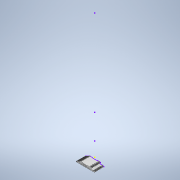
# Autodesk Inventor part: Pieza2
Saved by Autodesk Inventor 2021 (Build 250183000, 183)
## iProperties
Created: 2022-09-12
Part Number: Pieza2
Material: Genérico
Document SubType Name: Chapa
Designer: arthu
Density: 1 g/cm^3
Flat Pattern Width: 60 cm
Flat Pattern Length: 411.221 cm
Flat Pattern Area: 24673.3 cm^2
Sheet Metal Rule: Por defecto
Sheet Metal Width: 600.000 mm
Sheet Metal Length: 4112.213 mm
Sheet Metal Area: 2467327.803 mm^2
Appearance: Valor por defecto
Author: arthu
Autodesk Inventor part; units mm, degrees
(part 1 of 2)
ref_plane "YZ Plane" through (0, 0, 0) normal (1, 0, 0) x (0, 1, 0)
ref_plane "XZ Plane" through (0, 0, 0) normal (0, 1, 0) x (-1, 0, 0)
ref_plane "XY Plane" through (0, 0, 0) normal (0, 0, 1) x (1, 0, 0)
sketch "Boceto1" plane through (0, 0, 0) normal (0, 0, 1) x (1, 0, 0)
  line L0 (593.857, -227.2323) -> (593.8572, -227.2319)
  line L1 (533.5646, -194.9304) -> (533.5644, -194.9308)
  arc A0 (-280.9681, -73.3666) -> (280.9696, -73.3663) centre (0.0001, 907.6925) ccw
  arc A1 (-282.0694, -77.212) -> (282.0709, -77.2117) centre (0.0001, 907.6925) ccw
  line L2 (-378.2765, -109.4682) -> (-318.3462, -77.3608)
  line L3 (-376.3875, -112.9941) -> (-316.4572, -80.8866)
  arc A2 (373.059, -131.7091) -> (376.3889, -112.9936) centre (371.6669, -121.8075) ccw
  arc A3 (373.6159, -135.6702) -> (378.2779, -109.4677) centre (371.6669, -121.8075) ccw
  line L4 (378.2779, -109.4677) -> (318.3477, -77.3604)
  arc A4 (318.3477, -77.3604) -> (280.9696, -73.3663) centre (294.7357, -121.4335) ccw
  arc A5 (316.4587, -80.8863) -> (282.0709, -77.2117) centre (294.7357, -121.4335) ccw
  line L5 (376.3889, -112.9936) -> (316.4587, -80.8863)
  arc A6 (-393.407, -128.772) -> (373.059, -131.7091) centre (-0.011, 2521.9144) ccw
  arc A7 (-393.407, -128.772) -> (-424.3593, -134.1569) centre (-400.7473, -178.2302) ccw
  arc A8 (-393.9943, -132.7287) -> (373.6159, -135.6702) centre (-0.011, 2521.9144) ccw
  arc A9 (-393.9943, -132.7287) -> (-422.4704, -137.6828) centre (-400.7473, -178.2302) ccw
  line L6 (-485.1197, -166.709) -> (-424.3593, -134.1569)
  line L7 (-483.2307, -170.2349) -> (-422.4704, -137.6828)
  arc A10 (-483.2307, -170.2349) -> (-479.0854, -189.0324) centre (-478.5084, -179.0493) ccw
  arc A11 (-485.1197, -166.709) -> (-479.3162, -193.0257) centre (-478.5084, -179.0493) ccw
  arc A12 (-479.3162, -193.0257) -> (508.0847, -191.3269) centre (0.1136, 8102.2313) ccw
  arc A13 (-479.0854, -189.0324) -> (507.8402, -187.3344) centre (0.1136, 8102.2313) ccw
  line L8 (594.8017, -225.469) -> (534.5091, -193.1674)
  line L9 (592.9127, -228.9948) -> (532.6201, -196.6933)
  arc A14 (534.5091, -193.1674) -> (507.8402, -187.3344) centre (510.8969, -237.2409) ccw
  arc A15 (532.6201, -196.6933) -> (508.0847, -191.3269) centre (510.8969, -237.2409) ccw
  line L10 (-588.188, -247.8095) -> (588.1903, -247.8095)
  line L11 (588.1903, -251.8095) -> (400.752, -251.8095)
  arc A16 (588.1903, -247.8095) -> (592.9127, -228.9948) centre (588.1903, -237.8095) ccw
  arc A17 (588.1903, -251.8095) -> (594.8017, -225.469) centre (588.1903, -237.8095) ccw
  line L12 (-588.188, -251.8095) -> (588.1903, -251.8095)
  line L13 (-594.7994, -225.469) -> (-522.4838, -186.7262)
  line L14 (-592.9105, -228.9948) -> (-520.5949, -190.2521)
  arc A18 (-592.9105, -228.9948) -> (-588.188, -247.8095) centre (-588.188, -237.8095) ccw
  arc A19 (-594.7994, -225.469) -> (-588.188, -251.8095) centre (-588.188, -237.8095) ccw
  line L15 (-522.4838, -186.7262) -> (-520.5949, -190.2521)
  line L16 (-378.2765, -109.4682) -> (-376.3875, -112.9941)
  line L17 (0.0011, -247.8095) -> (0.0011, -251.8095)
  line L18 (-483.2307, -170.2349) -> (-485.1197, -166.709)
  line L19 (373.059, -131.7091) -> (373.6159, -135.6702)
  line L20 (268.9094, -80.8863) -> (268.0047, -76.987)
  arc A20 (-282.0694, -77.212) -> (-316.4572, -80.8866) centre (-294.7342, -121.4338) ccw
  arc A21 (-263.5915, -82.3174) -> (-333.7303, -90.1406) centre (-294.7342, -121.4338) ccw
  point P0 (0, 0)
  point P1 (280.9696, -73.3663)
  point P2 (282.0709, -77.2117)
  point P3 (373.059, -131.7091)
  point P4 (-424.3593, -134.1569)
  point P5 (508.0847, -191.3269)
  point P6 (-592.9105, -228.9948)
  point P7 (507.8402, -187.3344)
  point P8 (-422.4704, -137.6828)
  point P9 (378.2779, -109.4677)
  point P10 (-280.9681, -73.3666)
  constraints: 49 point on circle, 42 end point, 22 centre point, 22 tangent, 3 perpendicular, 2 coincident, 2 midpoint, 1 parallel, 1 point on line
extrude "Extrusión1" add sketch "Boceto1" along normal blind 600 contours A0 A4 L4 A3 L19 A2 L5 A5 A1 L20 | A8 A9 L7 L18 L6 A7 A6 L19 | A10 A13 A14 L8 A17 L11 L12 L17 L10 A16 L9 A15 A12 A11 L18 | L12 A19 L13 L15 L14 A18 L10 L17
extrude "Extrusión2" add sketch "Boceto1" along normal blind 600 contours A0 L20 A1 A21 | A21 A1 A20 L3 | A21 L3 L16 L2
sketch "Boceto2" plane through (318.3477, -77.3604, 600) normal (0.4722, 0.8815, 0) x (0.8815, -0.4722, 0)
  line L0 (0, 600) -> (67.989, 600) projected
  line L1 (67.989, 0) -> (81.9881, 0) projected
  line L2 (0, 600) -> (67.989, 600)
  line L3 (67.989, 600) -> (67.989, 0)
  line L4 (67.989, 0) -> (0, 0)
  line L5 (0, 0) -> (0, 600)
  line L6 (0, 600) -> (0, 0) projected
  line L7 (0, 600) -> (0, 300)
  line L8 (0, 300) -> (67.989, 300)
  line L9 (67.989, 600) -> (67.989, 0) projected
  ellipse E0 centre (33.9945, 300) end of major axis (51.9945, 300) minor radius 8
  ellipse E1 centre (33.9945, 332) end of major axis (51.9945, 332) minor radius 8
  ellipse E2 centre (33.9945, 364) end of major axis (51.9945, 364) minor radius 8
  ellipse E3 centre (33.9945, 396) end of major axis (51.9945, 396) minor radius 8
  ellipse E4 centre (33.9945, 428) end of major axis (51.9945, 428) minor radius 8
  ellipse E5 centre (33.9945, 460) end of major axis (51.9945, 460) minor radius 8
  ellipse E6 centre (33.9945, 492) end of major axis (51.9945, 492) minor radius 8
  ellipse E7 centre (33.9945, 524) end of major axis (51.9945, 524) minor radius 8
  ellipse E8 centre (33.9945, 556) end of major axis (51.9945, 556) minor radius 8
  ellipse E9 centre (33.9945, 268) end of major axis (51.9945, 268) minor radius 8
  ellipse E10 centre (33.9945, 300) end of major axis (51.9945, 300) minor radius 8
  ellipse E11 centre (33.9945, 332) end of major axis (51.9945, 332) minor radius 8
  ellipse E12 centre (33.9945, 364) end of major axis (51.9945, 364) minor radius 8
  ellipse E13 centre (33.9945, 396) end of major axis (51.9945, 396) minor radius 8
  ellipse E14 centre (33.9945, 428) end of major axis (51.9945, 428) minor radius 8
  ellipse E15 centre (33.9945, 460) end of major axis (51.9945, 460) minor radius 8
  ellipse E16 centre (33.9945, 492) end of major axis (51.9945, 492) minor radius 8
  ellipse E17 centre (33.9945, 524) end of major axis (51.9945, 524) minor radius 8
  ellipse E18 centre (33.9945, 236) end of major axis (51.9945, 236) minor radius 8
  ellipse E19 centre (33.9945, 268) end of major axis (51.9945, 268) minor radius 8
  ellipse E20 centre (33.9945, 300) end of major axis (51.9945, 300) minor radius 8
  ellipse E21 centre (33.9945, 332) end of major axis (51.9945, 332) minor radius 8
  ellipse E22 centre (33.9945, 364) end of major axis (51.9945, 364) minor radius 8
  ellipse E23 centre (33.9945, 396) end of major axis (51.9945, 396) minor radius 8
  ellipse E24 centre (33.9945, 428) end of major axis (51.9945, 428) minor radius 8
  ellipse E25 centre (33.9945, 460) end of major axis (51.9945, 460) minor radius 8
  ellipse E26 centre (33.9945, 492) end of major axis (51.9945, 492) minor radius 8
  ellipse E27 centre (33.9945, 204) end of major axis (51.9945, 204) minor radius 8
  ellipse E28 centre (33.9945, 236) end of major axis (51.9945, 236) minor radius 8
  ellipse E29 centre (33.9945, 268) end of major axis (51.9945, 268) minor radius 8
  ellipse E30 centre (33.9945, 300) end of major axis (51.9945, 300) minor radius 8
  ellipse E31 centre (33.9945, 332) end of major axis (51.9945, 332) minor radius 8
  ellipse E32 centre (33.9945, 364) end of major axis (51.9945, 364) minor radius 8
  ellipse E33 centre (33.9945, 396) end of major axis (51.9945, 396) minor radius 8
  ellipse E34 centre (33.9945, 428) end of major axis (51.9945, 428) minor radius 8
  ellipse E35 centre (33.9945, 460) end of major axis (51.9945, 460) minor radius 8
  ellipse E36 centre (33.9945, 172) end of major axis (51.9945, 172) minor radius 8
  ellipse E37 centre (33.9945, 204) end of major axis (51.9945, 204) minor radius 8
  ellipse E38 centre (33.9945, 236) end of major axis (51.9945, 236) minor radius 8
  ellipse E39 centre (33.9945, 268) end of major axis (51.9945, 268) minor radius 8
  ellipse E40 centre (33.9945, 300) end of major axis (51.9945, 300) minor radius 8
  ellipse E41 centre (33.9945, 332) end of major axis (51.9945, 332) minor radius 8
  ellipse E42 centre (33.9945, 364) end of major axis (51.9945, 364) minor radius 8
  ellipse E43 centre (33.9945, 396) end of major axis (51.9945, 396) minor radius 8
  ellipse E44 centre (33.9945, 428) end of major axis (51.9945, 428) minor radius 8
  ellipse E45 centre (33.9945, 140) end of major axis (51.9945, 140) minor radius 8
  ellipse E46 centre (33.9945, 172) end of major axis (51.9945, 172) minor radius 8
  ellipse E47 centre (33.9945, 204) end of major axis (51.9945, 204) minor radius 8
  ellipse E48 centre (33.9945, 236) end of major axis (51.9945, 236) minor radius 8
  ellipse E49 centre (33.9945, 268) end of major axis (51.9945, 268) minor radius 8
  ellipse E50 centre (33.9945, 300) end of major axis (51.9945, 300) minor radius 8
  ellipse E51 centre (33.9945, 332) end of major axis (51.9945, 332) minor radius 8
  ellipse E52 centre (33.9945, 364) end of major axis (51.9945, 364) minor radius 8
  ellipse E53 centre (33.9945, 396) end of major axis (51.9945, 396) minor radius 8
  ellipse E54 centre (33.9945, 108) end of major axis (51.9945, 108) minor radius 8
  ellipse E55 centre (33.9945, 140) end of major axis (51.9945, 140) minor radius 8
  ellipse E56 centre (33.9945, 172) end of major axis (51.9945, 172) minor radius 8
  ellipse E57 centre (33.9945, 204) end of major axis (51.9945, 204) minor radius 8
  ellipse E58 centre (33.9945, 236) end of major axis (51.9945, 236) minor radius 8
  ellipse E59 centre (33.9945, 268) end of major axis (51.9945, 268) minor radius 8
  ellipse E60 centre (33.9945, 300) end of major axis (51.9945, 300) minor radius 8
  ellipse E61 centre (33.9945, 332) end of major axis (51.9945, 332) minor radius 8
  ellipse E62 centre (33.9945, 364) end of major axis (51.9945, 364) minor radius 8
  ellipse E63 centre (33.9945, 76) end of major axis (51.9945, 76) minor radius 8
  ellipse E64 centre (33.9945, 108) end of major axis (51.9945, 108) minor radius 8
  ellipse E65 centre (33.9945, 140) end of major axis (51.9945, 140) minor radius 8
  ellipse E66 centre (33.9945, 172) end of major axis (51.9945, 172) minor radius 8
  ellipse E67 centre (33.9945, 204) end of major axis (51.9945, 204) minor radius 8
  ellipse E68 centre (33.9945, 236) end of major axis (51.9945, 236) minor radius 8
  ellipse E69 centre (33.9945, 268) end of major axis (51.9945, 268) minor radius 8
  ellipse E70 centre (33.9945, 300) end of major axis (51.9945, 300) minor radius 8
  ellipse E71 centre (33.9945, 332) end of major axis (51.9945, 332) minor radius 8
  ellipse E72 centre (33.9945, 44) end of major axis (51.9945, 44) minor radius 8
  ellipse E73 centre (33.9945, 76) end of major axis (51.9945, 76) minor radius 8
  ellipse E74 centre (33.9945, 108) end of major axis (51.9945, 108) minor radius 8
  ellipse E75 centre (33.9945, 140) end of major axis (51.9945, 140) minor radius 8
  ellipse E76 centre (33.9945, 172) end of major axis (51.9945, 172) minor radius 8
  ellipse E77 centre (33.9945, 204) end of major axis (51.9945, 204) minor radius 8
  ellipse E78 centre (33.9945, 236) end of major axis (51.9945, 236) minor radius 8
  ellipse E79 centre (33.9945, 268) end of major axis (51.9945, 268) minor radius 8
  ellipse E80 centre (33.9945, 300) end of major axis (51.9945, 300) minor radius 8
  line L10 (245.2285, 600) -> (221.0671, 600) projected
  line L11 (313.6287, 600) -> (313.6287, 0) projected
  line L12 (245.2285, 600) -> (313.6287, 600)
  line L13 (313.6287, 600) -> (313.6287, 0)
  line L14 (313.6287, 0) -> (245.2285, 0)
  line L15 (245.2285, 0) -> (245.2285, 600)
  line L16 (245.2285, 600) -> (245.2285, 0) projected
  line L17 (245.2285, 300) -> (313.6287, 300)
  ellipse E81 centre (279.4286, 300) end of major axis (297.4286, 300) minor radius 8
  ellipse E82 centre (279.4286, 332) end of major axis (297.4286, 332) minor radius 8
  ellipse E83 centre (279.4286, 364) end of major axis (297.4286, 364) minor radius 8
  ellipse E84 centre (279.4286, 396) end of major axis (297.4286, 396) minor radius 8
  ellipse E85 centre (279.4286, 428) end of major axis (297.4286, 428) minor radius 8
  ellipse E86 centre (279.4286, 460) end of major axis (297.4286, 460) minor radius 8
  ellipse E87 centre (279.4286, 492) end of major axis (297.4286, 492) minor radius 8
  ellipse E88 centre (279.4286, 524) end of major axis (297.4286, 524) minor radius 8
  ellipse E89 centre (279.4286, 556) end of major axis (297.4286, 556) minor radius 8
  ellipse E90 centre (279.4286, 268) end of major axis (297.4286, 268) minor radius 8
  ellipse E91 centre (279.4286, 300) end of major axis (297.4286, 300) minor radius 8
  ellipse E92 centre (279.4286, 332) end of major axis (297.4286, 332) minor radius 8
  ellipse E93 centre (279.4286, 364) end of major axis (297.4286, 364) minor radius 8
  ellipse E94 centre (279.4286, 396) end of major axis (297.4286, 396) minor radius 8
  ellipse E95 centre (279.4286, 428) end of major axis (297.4286, 428) minor radius 8
  ellipse E96 centre (279.4286, 460) end of major axis (297.4286, 460) minor radius 8
  ellipse E97 centre (279.4286, 492) end of major axis (297.4286, 492) minor radius 8
  ellipse E98 centre (279.4286, 524) end of major axis (297.4286, 524) minor radius 8
  ellipse E99 centre (279.4286, 236) end of major axis (297.4286, 236) minor radius 8
  ellipse E100 centre (279.4286, 268) end of major axis (297.4286, 268) minor radius 8
  ellipse E101 centre (279.4286, 300) end of major axis (297.4286, 300) minor radius 8
  ellipse E102 centre (279.4286, 332) end of major axis (297.4286, 332) minor radius 8
  ellipse E103 centre (279.4286, 364) end of major axis (297.4286, 364) minor radius 8
  ellipse E104 centre (279.4286, 396) end of major axis (297.4286, 396) minor radius 8
  ellipse E105 centre (279.4286, 428) end of major axis (297.4286, 428) minor radius 8
  ellipse E106 centre (279.4286, 460) end of major axis (297.4286, 460) minor radius 8
  ellipse E107 centre (279.4286, 492) end of major axis (297.4286, 492) minor radius 8
  ellipse E108 centre (279.4286, 204) end of major axis (297.4286, 204) minor radius 8
  ellipse E109 centre (279.4286, 236) end of major axis (297.4286, 236) minor radius 8
  ellipse E110 centre (279.4286, 268) end of major axis (297.4286, 268) minor radius 8
  ellipse E111 centre (279.4286, 300) end of major axis (297.4286, 300) minor radius 8
  ellipse E112 centre (279.4286, 332) end of major axis (297.4286, 332) minor radius 8
  ellipse E113 centre (279.4286, 364) end of major axis (297.4286, 364) minor radius 8
  ellipse E114 centre (279.4286, 396) end of major axis (297.4286, 396) minor radius 8
  ellipse E115 centre (279.4286, 428) end of major axis (297.4286, 428) minor radius 8
  ellipse E116 centre (279.4286, 460) end of major axis (297.4286, 460) minor radius 8
  ellipse E117 centre (279.4286, 172) end of major axis (297.4286, 172) minor radius 8
  ellipse E118 centre (279.4286, 204) end of major axis (297.4286, 204) minor radius 8
  ellipse E119 centre (279.4286, 236) end of major axis (297.4286, 236) minor radius 8
  ellipse E120 centre (279.4286, 268) end of major axis (297.4286, 268) minor radius 8
  ellipse E121 centre (279.4286, 300) end of major axis (297.4286, 300) minor radius 8
  ellipse E122 centre (279.4286, 332) end of major axis (297.4286, 332) minor radius 8
  ellipse E123 centre (279.4286, 364) end of major axis (297.4286, 364) minor radius 8
  ellipse E124 centre (279.4286, 396) end of major axis (297.4286, 396) minor radius 8
  ellipse E125 centre (279.4286, 428) end of major axis (297.4286, 428) minor radius 8
  ellipse E126 centre (279.4286, 140) end of major axis (297.4286, 140) minor radius 8
  ellipse E127 centre (279.4286, 172) end of major axis (297.4286, 172) minor radius 8
  ellipse E128 centre (279.4286, 204) end of major axis (297.4286, 204) minor radius 8
  ellipse E129 centre (279.4286, 236) end of major axis (297.4286, 236) minor radius 8
  ellipse E130 centre (279.4286, 268) end of major axis (297.4286, 268) minor radius 8
  ellipse E131 centre (279.4286, 300) end of major axis (297.4286, 300) minor radius 8
  ellipse E132 centre (279.4286, 332) end of major axis (297.4286, 332) minor radius 8
  ellipse E133 centre (279.4286, 364) end of major axis (297.4286, 364) minor radius 8
  ellipse E134 centre (279.4286, 396) end of major axis (297.4286, 396) minor radius 8
  ellipse E135 centre (279.4286, 108) end of major axis (297.4286, 108) minor radius 8
  ellipse E136 centre (279.4286, 140) end of major axis (297.4286, 140) minor radius 8
  ellipse E137 centre (279.4286, 172) end of major axis (297.4286, 172) minor radius 8
  ellipse E138 centre (279.4286, 204) end of major axis (297.4286, 204) minor radius 8
  ellipse E139 centre (279.4286, 236) end of major axis (297.4286, 236) minor radius 8
  ellipse E140 centre (279.4286, 268) end of major axis (297.4286, 268) minor radius 8
  ellipse E141 centre (279.4286, 300) end of major axis (297.4286, 300) minor radius 8
  ellipse E142 centre (279.4286, 332) end of major axis (297.4286, 332) minor radius 8
  ellipse E143 centre (279.4286, 364) end of major axis (297.4286, 364) minor radius 8
  ellipse E144 centre (279.4286, 76) end of major axis (297.4286, 76) minor radius 8
  ellipse E145 centre (279.4286, 108) end of major axis (297.4286, 108) minor radius 8
  ellipse E146 centre (279.4286, 140) end of major axis (297.4286, 140) minor radius 8
  ellipse E147 centre (279.4286, 172) end of major axis (297.4286, 172) minor radius 8
  ellipse E148 centre (279.4286, 204) end of major axis (297.4286, 204) minor radius 8
  ellipse E149 centre (279.4286, 236) end of major axis (297.4286, 236) minor radius 8
  ellipse E150 centre (279.4286, 268) end of major axis (297.4286, 268) minor radius 8
  ellipse E151 centre (279.4286, 300) end of major axis (297.4286, 300) minor radius 8
  ellipse E152 centre (279.4286, 332) end of major axis (297.4286, 332) minor radius 8
  ellipse E153 centre (279.4286, 44) end of major axis (297.4286, 44) minor radius 8
  ellipse E154 centre (279.4286, 76) end of major axis (297.4286, 76) minor radius 8
  ellipse E155 centre (279.4286, 108) end of major axis (297.4286, 108) minor radius 8
  ellipse E156 centre (279.4286, 140) end of major axis (297.4286, 140) minor radius 8
  ellipse E157 centre (279.4286, 172) end of major axis (297.4286, 172) minor radius 8
  ellipse E158 centre (279.4286, 204) end of major axis (297.4286, 204) minor radius 8
  ellipse E159 centre (279.4286, 236) end of major axis (297.4286, 236) minor radius 8
  ellipse E160 centre (279.4286, 268) end of major axis (297.4286, 268) minor radius 8
  ellipse E161 centre (279.4286, 300) end of major axis (297.4286, 300) minor radius 8
  point P0 (-317.1463, 600)
  point P1 (76.2536, 0)
  point P2 (279.4286, 308)
  point P3 (279.4286, 292)
  point P4 (33.9945, 308)
  point P5 (33.9945, 292)
  point P6 (279.4286, 340)
  point P7 (279.4286, 324)
  point P8 (279.4286, 372)
  point P9 (279.4286, 356)
  point P10 (279.4286, 404)
  point P11 (279.4286, 388)
  point P12 (279.4286, 436)
  point P13 (279.4286, 420)
  point P14 (279.4286, 468)
  point P15 (279.4286, 452)
  point P16 (279.4286, 500)
  point P17 (279.4286, 484)
  point P18 (279.4286, 532)
  point P19 (279.4286, 516)
  point P20 (279.4286, 564)
  point P21 (279.4286, 548)
  point P22 (279.4286, 276)
  point P23 (279.4286, 260)
  point P24 (279.4286, 308)
  point P25 (279.4286, 292)
  point P26 (279.4286, 340)
  point P27 (279.4286, 324)
  point P28 (279.4286, 372)
  point P29 (279.4286, 356)
  point P30 (279.4286, 404)
  point P31 (279.4286, 388)
  point P32 (279.4286, 436)
  point P33 (279.4286, 420)
  point P34 (279.4286, 468)
  point P35 (279.4286, 452)
  point P36 (279.4286, 500)
  point P37 (279.4286, 484)
  point P38 (279.4286, 532)
  point P39 (279.4286, 516)
  point P40 (279.4286, 244)
  point P41 (279.4286, 228)
  point P42 (279.4286, 276)
  point P43 (279.4286, 260)
  point P44 (279.4286, 308)
  point P45 (279.4286, 292)
  point P46 (279.4286, 340)
  point P47 (279.4286, 324)
  point P48 (279.4286, 372)
  point P49 (279.4286, 356)
  point P50 (279.4286, 404)
  point P51 (279.4286, 388)
  point P52 (279.4286, 436)
  point P53 (279.4286, 420)
  point P54 (279.4286, 468)
  point P55 (279.4286, 452)
  point P56 (279.4286, 500)
  point P57 (279.4286, 484)
  point P58 (279.4286, 212)
  point P59 (279.4286, 196)
  point P60 (279.4286, 244)
  point P61 (279.4286, 228)
  point P62 (279.4286, 276)
  point P63 (279.4286, 260)
  point P64 (279.4286, 308)
  point P65 (279.4286, 292)
  point P66 (279.4286, 340)
  point P67 (279.4286, 324)
  point P68 (279.4286, 372)
  point P69 (279.4286, 356)
  point P70 (279.4286, 404)
  point P71 (279.4286, 388)
  point P72 (279.4286, 436)
  point P73 (279.4286, 420)
  point P74 (279.4286, 468)
  point P75 (279.4286, 452)
  point P76 (279.4286, 180)
  point P77 (279.4286, 164)
  point P78 (279.4286, 212)
  point P79 (279.4286, 196)
  point P80 (279.4286, 244)
  point P81 (279.4286, 228)
  point P82 (279.4286, 276)
  point P83 (279.4286, 260)
  point P84 (279.4286, 308)
  point P85 (279.4286, 292)
  point P86 (279.4286, 340)
  point P87 (279.4286, 324)
  point P88 (279.4286, 372)
  point P89 (279.4286, 356)
  point P90 (279.4286, 404)
  point P91 (279.4286, 388)
  point P92 (279.4286, 436)
  point P93 (279.4286, 420)
  point P94 (279.4286, 148)
  point P95 (279.4286, 132)
  point P96 (279.4286, 180)
  point P97 (279.4286, 164)
  point P98 (279.4286, 212)
  point P99 (279.4286, 196)
  point P100 (279.4286, 244)
  point P101 (279.4286, 228)
  point P102 (279.4286, 276)
  point P103 (279.4286, 260)
  point P104 (279.4286, 308)
  point P105 (279.4286, 292)
  point P106 (279.4286, 340)
  point P107 (279.4286, 324)
  point P108 (279.4286, 372)
  point P109 (279.4286, 356)
  point P110 (279.4286, 404)
  point P111 (279.4286, 388)
  point P112 (279.4286, 116)
  point P113 (279.4286, 100)
  point P114 (279.4286, 148)
  point P115 (279.4286, 132)
  point P116 (279.4286, 180)
  point P117 (279.4286, 164)
  point P118 (279.4286, 212)
  point P119 (279.4286, 196)
  point P120 (279.4286, 244)
  point P121 (279.4286, 228)
  point P122 (279.4286, 276)
  point P123 (279.4286, 260)
  point P124 (279.4286, 308)
  point P125 (279.4286, 292)
  point P126 (279.4286, 340)
  point P127 (279.4286, 324)
  point P128 (279.4286, 372)
  point P129 (279.4286, 356)
  point P130 (279.4286, 84)
  point P131 (279.4286, 68)
  point P132 (279.4286, 116)
  point P133 (279.4286, 100)
  point P134 (279.4286, 148)
  point P135 (279.4286, 132)
  point P136 (279.4286, 180)
  point P137 (279.4286, 164)
  point P138 (279.4286, 212)
  point P139 (279.4286, 196)
  point P140 (279.4286, 244)
  point P141 (279.4286, 228)
  point P142 (279.4286, 276)
  point P143 (279.4286, 260)
  point P144 (279.4286, 308)
  point P145 (279.4286, 292)
  point P146 (279.4286, 340)
  point P147 (279.4286, 324)
  point P148 (279.4286, 52)
  point P149 (279.4286, 36)
  point P150 (279.4286, 84)
  point P151 (279.4286, 68)
  point P152 (279.4286, 116)
  point P153 (279.4286, 100)
  point P154 (279.4286, 148)
  point P155 (279.4286, 132)
  point P156 (279.4286, 180)
  point P157 (279.4286, 164)
  point P158 (279.4286, 212)
  point P159 (279.4286, 196)
  point P160 (279.4286, 244)
  point P161 (279.4286, 228)
  point P162 (279.4286, 276)
  point P163 (279.4286, 260)
  point P164 (279.4286, 308)
  point P165 (279.4286, 292)
  dimension "d46" = 18
  dimension "d35" = 300
  dimension "d36" = 90
  dimension "d37" = 18
  dimension "d40" = 32
  dimension "d43" = 32
  dimension "d47" = 16
  dimension "d49" = 16
  dimension "d52" = 32
  dimension "d55" = 32
  constraints: 84 vertical, 80 centre point, 22 end point, 6 midpoint, 4 parallel, 2 horizontal, 2 perpendicular, 728 other
  measures "d35" distance of L0.start L7.end
  measures "d36" angle of L8 L7
  measures "d40" distance of E0.centre E1.centre
  measures "d43" distance of E0.centre E9.centre
  measures "d47" distance of point (279.429, 292) point (279.429, 308)
  measures "d49" distance of point (33.995, 308) point (33.995, 292)
  measures "d52" distance of point (279.429, 300) point (279.429, 332)
  measures "d55" distance of point (279.429, 300) point (279.429, 268)
extrude "Extrusión3" cut sketch "Boceto2" against normal mid plane 10 contours E81 L17 | L17 E81 | E82 | E83 | E84 | E85 | E86 | E87 | E88 | E89 | E90 | E99 | E108 | E117 | E126 | E135 | E144 | E153
extrude "Extrusión4" cut sketch "Boceto2" along normal mid plane 32.5 contours E0 L8 | L8 E0 | E1 | E2 | E3 | E4 | E5 | E6 | E7 | E8 | E9 | E18 | E27 | E36 | E45 | E54 | E63 | E72
sketch "Boceto3" plane through (-378.2765, -109.4682, 600) normal (-0.4722, 0.8815, 0) x (0.8815, 0.4722, 0)
  line L0 (67.9892, 600) -> (67.9892, 0) projected
  line L1 (0, 600) -> (0, 0) projected
  line L2 (67.9892, 0) -> (0, 0)
  line L3 (0, 0) -> (0, 600)
  line L4 (0, 600) -> (67.9892, 600)
  line L5 (67.9892, 600) -> (67.9892, 0)
  line L6 (67.9892, 300) -> (0, 300)
  ellipse E0 centre (33.9946, 300) end of major axis (15.9946, 300) minor radius 8
  ellipse E1 centre (33.9946, 268) end of major axis (15.9946, 268) minor radius 8
  ellipse E2 centre (33.9946, 236) end of major axis (15.9946, 236) minor radius 8
  ellipse E3 centre (33.9946, 204) end of major axis (15.9946, 204) minor radius 8
  ellipse E4 centre (33.9946, 172) end of major axis (15.9946, 172) minor radius 8
  ellipse E5 centre (33.9946, 140) end of major axis (15.9946, 140) minor radius 8
  ellipse E6 centre (33.9946, 108) end of major axis (15.9946, 108) minor radius 8
  ellipse E7 centre (33.9946, 76) end of major axis (15.9946, 76) minor radius 8
  ellipse E8 centre (33.9946, 44) end of major axis (15.9946, 44) minor radius 8
  ellipse E9 centre (33.9946, 332) end of major axis (15.9946, 332) minor radius 8
  ellipse E10 centre (33.9946, 300) end of major axis (15.9946, 300) minor radius 8
  ellipse E11 centre (33.9946, 268) end of major axis (15.9946, 268) minor radius 8
  ellipse E12 centre (33.9946, 236) end of major axis (15.9946, 236) minor radius 8
  ellipse E13 centre (33.9946, 204) end of major axis (15.9946, 204) minor radius 8
  ellipse E14 centre (33.9946, 172) end of major axis (15.9946, 172) minor radius 8
  ellipse E15 centre (33.9946, 140) end of major axis (15.9946, 140) minor radius 8
  ellipse E16 centre (33.9946, 108) end of major axis (15.9946, 108) minor radius 8
  ellipse E17 centre (33.9946, 76) end of major axis (15.9946, 76) minor radius 8
  ellipse E18 centre (33.9946, 364) end of major axis (15.9946, 364) minor radius 8
  ellipse E19 centre (33.9946, 332) end of major axis (15.9946, 332) minor radius 8
  ellipse E20 centre (33.9946, 300) end of major axis (15.9946, 300) minor radius 8
  ellipse E21 centre (33.9946, 268) end of major axis (15.9946, 268) minor radius 8
  ellipse E22 centre (33.9946, 236) end of major axis (15.9946, 236) minor radius 8
  ellipse E23 centre (33.9946, 204) end of major axis (15.9946, 204) minor radius 8
  ellipse E24 centre (33.9946, 172) end of major axis (15.9946, 172) minor radius 8
  ellipse E25 centre (33.9946, 140) end of major axis (15.9946, 140) minor radius 8
  ellipse E26 centre (33.9946, 108) end of major axis (15.9946, 108) minor radius 8
  ellipse E27 centre (33.9946, 396) end of major axis (15.9946, 396) minor radius 8
  ellipse E28 centre (33.9946, 364) end of major axis (15.9946, 364) minor radius 8
  ellipse E29 centre (33.9946, 332) end of major axis (15.9946, 332) minor radius 8
  ellipse E30 centre (33.9946, 300) end of major axis (15.9946, 300) minor radius 8
  ellipse E31 centre (33.9946, 268) end of major axis (15.9946, 268) minor radius 8
  ellipse E32 centre (33.9946, 236) end of major axis (15.9946, 236) minor radius 8
  ellipse E33 centre (33.9946, 204) end of major axis (15.9946, 204) minor radius 8
  ellipse E34 centre (33.9946, 172) end of major axis (15.9946, 172) minor radius 8
  ellipse E35 centre (33.9946, 140) end of major axis (15.9946, 140) minor radius 8
  ellipse E36 centre (33.9946, 428) end of major axis (15.9946, 428) minor radius 8
  ellipse E37 centre (33.9946, 396) end of major axis (15.9946, 396) minor radius 8
  ellipse E38 centre (33.9946, 364) end of major axis (15.9946, 364) minor radius 8
  ellipse E39 centre (33.9946, 332) end of major axis (15.9946, 332) minor radius 8
  ellipse E40 centre (33.9946, 300) end of major axis (15.9946, 300) minor radius 8
  ellipse E41 centre (33.9946, 268) end of major axis (15.9946, 268) minor radius 8
  ellipse E42 centre (33.9946, 236) end of major axis (15.9946, 236) minor radius 8
  ellipse E43 centre (33.9946, 204) end of major axis (15.9946, 204) minor radius 8
  ellipse E44 centre (33.9946, 172) end of major axis (15.9946, 172) minor radius 8
  ellipse E45 centre (33.9946, 460) end of major axis (15.9946, 460) minor radius 8
  ellipse E46 centre (33.9946, 428) end of major axis (15.9946, 428) minor radius 8
  ellipse E47 centre (33.9946, 396) end of major axis (15.9946, 396) minor radius 8
  ellipse E48 centre (33.9946, 364) end of major axis (15.9946, 364) minor radius 8
  ellipse E49 centre (33.9946, 332) end of major axis (15.9946, 332) minor radius 8
  ellipse E50 centre (33.9946, 300) end of major axis (15.9946, 300) minor radius 8
  ellipse E51 centre (33.9946, 268) end of major axis (15.9946, 268) minor radius 8
  ellipse E52 centre (33.9946, 236) end of major axis (15.9946, 236) minor radius 8
  ellipse E53 centre (33.9946, 204) end of major axis (15.9946, 204) minor radius 8
  ellipse E54 centre (33.9946, 492) end of major axis (15.9946, 492) minor radius 8
  ellipse E55 centre (33.9946, 460) end of major axis (15.9946, 460) minor radius 8
  ellipse E56 centre (33.9946, 428) end of major axis (15.9946, 428) minor radius 8
  ellipse E57 centre (33.9946, 396) end of major axis (15.9946, 396) minor radius 8
  ellipse E58 centre (33.9946, 364) end of major axis (15.9946, 364) minor radius 8
  ellipse E59 centre (33.9946, 332) end of major axis (15.9946, 332) minor radius 8
  ellipse E60 centre (33.9946, 300) end of major axis (15.9946, 300) minor radius 8
  ellipse E61 centre (33.9946, 268) end of major axis (15.9946, 268) minor radius 8
  ellipse E62 centre (33.9946, 236) end of major axis (15.9946, 236) minor radius 8
  ellipse E63 centre (33.9946, 524) end of major axis (15.9946, 524) minor radius 8
  ellipse E64 centre (33.9946, 492) end of major axis (15.9946, 492) minor radius 8
  ellipse E65 centre (33.9946, 460) end of major axis (15.9946, 460) minor radius 8
  ellipse E66 centre (33.9946, 428) end of major axis (15.9946, 428) minor radius 8
  ellipse E67 centre (33.9946, 396) end of major axis (15.9946, 396) minor radius 8
  ellipse E68 centre (33.9946, 364) end of major axis (15.9946, 364) minor radius 8
  ellipse E69 centre (33.9946, 332) end of major axis (15.9946, 332) minor radius 8
  ellipse E70 centre (33.9946, 300) end of major axis (15.9946, 300) minor radius 8
  ellipse E71 centre (33.9946, 268) end of major axis (15.9946, 268) minor radius 8
  ellipse E72 centre (33.9946, 556) end of major axis (15.9946, 556) minor radius 8
  ellipse E73 centre (33.9946, 524) end of major axis (15.9946, 524) minor radius 8
  ellipse E74 centre (33.9946, 492) end of major axis (15.9946, 492) minor radius 8
  ellipse E75 centre (33.9946, 460) end of major axis (15.9946, 460) minor radius 8
  ellipse E76 centre (33.9946, 428) end of major axis (15.9946, 428) minor radius 8
  ellipse E77 centre (33.9946, 396) end of major axis (15.9946, 396) minor radius 8
  ellipse E78 centre (33.9946, 364) end of major axis (15.9946, 364) minor radius 8
  ellipse E79 centre (33.9946, 332) end of major axis (15.9946, 332) minor radius 8
  ellipse E80 centre (33.9946, 300) end of major axis (15.9946, 300) minor radius 8
  line L7 (-52.2796, 600) -> (-52.2796, 0) projected
  line L8 (-135.2102, 600) -> (-121.2104, 600) projected
  line L9 (-52.2796, 0) -> (-121.2104, 0)
  line L10 (-121.2104, 0) -> (-121.2104, 600)
  line L11 (-121.2104, 600) -> (-52.2796, 600)
  line L12 (-52.2796, 600) -> (-52.2796, 0)
  line L13 (-52.2796, 300) -> (-121.2104, 300)
  line L14 (-121.2104, 600) -> (-121.2104, 0) projected
  ellipse E81 centre (-86.745, 300) end of major axis (-104.745, 300) minor radius 8
  ellipse E82 centre (-86.745, 268) end of major axis (-104.745, 268) minor radius 8
  ellipse E83 centre (-86.745, 236) end of major axis (-104.745, 236) minor radius 8
  ellipse E84 centre (-86.745, 204) end of major axis (-104.745, 204) minor radius 8
  ellipse E85 centre (-86.745, 172) end of major axis (-104.745, 172) minor radius 8
  ellipse E86 centre (-86.745, 140) end of major axis (-104.745, 140) minor radius 8
  ellipse E87 centre (-86.745, 108) end of major axis (-104.745, 108) minor radius 8
  ellipse E88 centre (-86.745, 76) end of major axis (-104.745, 76) minor radius 8
  ellipse E89 centre (-86.745, 44) end of major axis (-104.745, 44) minor radius 8
  ellipse E90 centre (-86.745, 332) end of major axis (-104.745, 332) minor radius 8
  ellipse E91 centre (-86.745, 300) end of major axis (-104.745, 300) minor radius 8
  ellipse E92 centre (-86.745, 268) end of major axis (-104.745, 268) minor radius 8
  ellipse E93 centre (-86.745, 236) end of major axis (-104.745, 236) minor radius 8
  ellipse E94 centre (-86.745, 204) end of major axis (-104.745, 204) minor radius 8
  ellipse E95 centre (-86.745, 172) end of major axis (-104.745, 172) minor radius 8
  ellipse E96 centre (-86.745, 140) end of major axis (-104.745, 140) minor radius 8
  ellipse E97 centre (-86.745, 108) end of major axis (-104.745, 108) minor radius 8
  ellipse E98 centre (-86.745, 76) end of major axis (-104.745, 76) minor radius 8
  ellipse E99 centre (-86.745, 364) end of major axis (-104.745, 364) minor radius 8
  ellipse E100 centre (-86.745, 332) end of major axis (-104.745, 332) minor radius 8
  ellipse E101 centre (-86.745, 300) end of major axis (-104.745, 300) minor radius 8
  ellipse E102 centre (-86.745, 268) end of major axis (-104.745, 268) minor radius 8
  ellipse E103 centre (-86.745, 236) end of major axis (-104.745, 236) minor radius 8
  ellipse E104 centre (-86.745, 204) end of major axis (-104.745, 204) minor radius 8
  ellipse E105 centre (-86.745, 172) end of major axis (-104.745, 172) minor radius 8
  ellipse E106 centre (-86.745, 140) end of major axis (-104.745, 140) minor radius 8
  ellipse E107 centre (-86.745, 108) end of major axis (-104.745, 108) minor radius 8
  ellipse E108 centre (-86.745, 396) end of major axis (-104.745, 396) minor radius 8
  ellipse E109 centre (-86.745, 364) end of major axis (-104.745, 364) minor radius 8
  ellipse E110 centre (-86.745, 332) end of major axis (-104.745, 332) minor radius 8
  ellipse E111 centre (-86.745, 300) end of major axis (-104.745, 300) minor radius 8
  ellipse E112 centre (-86.745, 268) end of major axis (-104.745, 268) minor radius 8
  ellipse E113 centre (-86.745, 236) end of major axis (-104.745, 236) minor radius 8
  ellipse E114 centre (-86.745, 204) end of major axis (-104.745, 204) minor radius 8
  ellipse E115 centre (-86.745, 172) end of major axis (-104.745, 172) minor radius 8
  ellipse E116 centre (-86.745, 140) end of major axis (-104.745, 140) minor radius 8
  ellipse E117 centre (-86.745, 428) end of major axis (-104.745, 428) minor radius 8
  ellipse E118 centre (-86.745, 396) end of major axis (-104.745, 396) minor radius 8
  ellipse E119 centre (-86.745, 364) end of major axis (-104.745, 364) minor radius 8
  ellipse E120 centre (-86.745, 332) end of major axis (-104.745, 332) minor radius 8
  ellipse E121 centre (-86.745, 300) end of major axis (-104.745, 300) minor radius 8
  ellipse E122 centre (-86.745, 268) end of major axis (-104.745, 268) minor radius 8
  ellipse E123 centre (-86.745, 236) end of major axis (-104.745, 236) minor radius 8
  ellipse E124 centre (-86.745, 204) end of major axis (-104.745, 204) minor radius 8
  ellipse E125 centre (-86.745, 172) end of major axis (-104.745, 172) minor radius 8
  ellipse E126 centre (-86.745, 460) end of major axis (-104.745, 460) minor radius 8
  ellipse E127 centre (-86.745, 428) end of major axis (-104.745, 428) minor radius 8
  ellipse E128 centre (-86.745, 396) end of major axis (-104.745, 396) minor radius 8
  ellipse E129 centre (-86.745, 364) end of major axis (-104.745, 364) minor radius 8
  ellipse E130 centre (-86.745, 332) end of major axis (-104.745, 332) minor radius 8
  ellipse E131 centre (-86.745, 300) end of major axis (-104.745, 300) minor radius 8
  ellipse E132 centre (-86.745, 268) end of major axis (-104.745, 268) minor radius 8
  ellipse E133 centre (-86.745, 236) end of major axis (-104.745, 236) minor radius 8
  ellipse E134 centre (-86.745, 204) end of major axis (-104.745, 204) minor radius 8
  ellipse E135 centre (-86.745, 492) end of major axis (-104.745, 492) minor radius 8
  ellipse E136 centre (-86.745, 460) end of major axis (-104.745, 460) minor radius 8
  ellipse E137 centre (-86.745, 428) end of major axis (-104.745, 428) minor radius 8
  ellipse E138 centre (-86.745, 396) end of major axis (-104.745, 396) minor radius 8
  ellipse E139 centre (-86.745, 364) end of major axis (-104.745, 364) minor radius 8
  ellipse E140 centre (-86.745, 332) end of major axis (-104.745, 332) minor radius 8
  ellipse E141 centre (-86.745, 300) end of major axis (-104.745, 300) minor radius 8
  ellipse E142 centre (-86.745, 268) end of major axis (-104.745, 268) minor radius 8
  ellipse E143 centre (-86.745, 236) end of major axis (-104.745, 236) minor radius 8
  ellipse E144 centre (-86.745, 524) end of major axis (-104.745, 524) minor radius 8
  ellipse E145 centre (-86.745, 492) end of major axis (-104.745, 492) minor radius 8
  ellipse E146 centre (-86.745, 460) end of major axis (-104.745, 460) minor radius 8
  ellipse E147 centre (-86.745, 428) end of major axis (-104.745, 428) minor radius 8
  ellipse E148 centre (-86.745, 396) end of major axis (-104.745, 396) minor radius 8
  ellipse E149 centre (-86.745, 364) end of major axis (-104.745, 364) minor radius 8
  ellipse E150 centre (-86.745, 332) end of major axis (-104.745, 332) minor radius 8
  ellipse E151 centre (-86.745, 300) end of major axis (-104.745, 300) minor radius 8
  ellipse E152 centre (-86.745, 268) end of major axis (-104.745, 268) minor radius 8
  ellipse E153 centre (-86.745, 556) end of major axis (-104.745, 556) minor radius 8
  ellipse E154 centre (-86.745, 524) end of major axis (-104.745, 524) minor radius 8
  ellipse E155 centre (-86.745, 492) end of major axis (-104.745, 492) minor radius 8
  ellipse E156 centre (-86.745, 460) end of major axis (-104.745, 460) minor radius 8
  ellipse E157 centre (-86.745, 428) end of major axis (-104.745, 428) minor radius 8
  ellipse E158 centre (-86.745, 396) end of major axis (-104.745, 396) minor radius 8
  ellipse E159 centre (-86.745, 364) end of major axis (-104.745, 364) minor radius 8
  ellipse E160 centre (-86.745, 332) end of major axis (-104.745, 332) minor radius 8
  ellipse E161 centre (-86.745, 300) end of major axis (-104.745, 300) minor radius 8
  line L15 (-163.5987, 600) -> (-163.5987, 0) projected
  line L16 (-245.6387, 600) -> (-245.6387, 0) projected
  line L17 (-163.5987, 0) -> (-245.6387, 0)
  line L18 (-245.6387, 0) -> (-245.6387, 600)
  line L19 (-245.6387, 600) -> (-163.5987, 600)
  line L20 (-163.5987, 600) -> (-163.5987, 0)
  line L21 (-163.5987, 300) -> (-245.6387, 300)
  ellipse E162 centre (-204.6187, 300) end of major axis (-222.6187, 300) minor radius 8
  ellipse E163 centre (-204.6187, 268) end of major axis (-222.6187, 268) minor radius 8
  ellipse E164 centre (-204.6187, 236) end of major axis (-222.6187, 236) minor radius 8
  ellipse E165 centre (-204.6187, 204) end of major axis (-222.6187, 204) minor radius 8
  ellipse E166 centre (-204.6187, 172) end of major axis (-222.6187, 172) minor radius 8
  ellipse E167 centre (-204.6187, 140) end of major axis (-222.6187, 140) minor radius 8
  ellipse E168 centre (-204.6187, 108) end of major axis (-222.6187, 108) minor radius 8
  ellipse E169 centre (-204.6187, 76) end of major axis (-222.6187, 76) minor radius 8
  ellipse E170 centre (-204.6187, 44) end of major axis (-222.6187, 44) minor radius 8
  ellipse E171 centre (-204.6187, 332) end of major axis (-222.6187, 332) minor radius 8
  ellipse E172 centre (-204.6187, 300) end of major axis (-222.6187, 300) minor radius 8
  ellipse E173 centre (-204.6187, 268) end of major axis (-222.6187, 268) minor radius 8
  ellipse E174 centre (-204.6187, 236) end of major axis (-222.6187, 236) minor radius 8
  ellipse E175 centre (-204.6187, 204) end of major axis (-222.6187, 204) minor radius 8
  ellipse E176 centre (-204.6187, 172) end of major axis (-222.6187, 172) minor radius 8
  ellipse E177 centre (-204.6187, 140) end of major axis (-222.6187, 140) minor radius 8
  ellipse E178 centre (-204.6187, 108) end of major axis (-222.6187, 108) minor radius 8
  ellipse E179 centre (-204.6187, 76) end of major axis (-222.6187, 76) minor radius 8
  ellipse E180 centre (-204.6187, 364) end of major axis (-222.6187, 364) minor radius 8
  ellipse E181 centre (-204.6187, 332) end of major axis (-222.6187, 332) minor radius 8
  ellipse E182 centre (-204.6187, 300) end of major axis (-222.6187, 300) minor radius 8
  ellipse E183 centre (-204.6187, 268) end of major axis (-222.6187, 268) minor radius 8
  ellipse E184 centre (-204.6187, 236) end of major axis (-222.6187, 236) minor radius 8
  ellipse E185 centre (-204.6187, 204) end of major axis (-222.6187, 204) minor radius 8
  ellipse E186 centre (-204.6187, 172) end of major axis (-222.6187, 172) minor radius 8
  ellipse E187 centre (-204.6187, 140) end of major axis (-222.6187, 140) minor radius 8
  ellipse E188 centre (-204.6187, 108) end of major axis (-222.6187, 108) minor radius 8
  ellipse E189 centre (-204.6187, 396) end of major axis (-222.6187, 396) minor radius 8
  ellipse E190 centre (-204.6187, 364) end of major axis (-222.6187, 364) minor radius 8
  ellipse E191 centre (-204.6187, 332) end of major axis (-222.6187, 332) minor radius 8
  ellipse E192 centre (-204.6187, 300) end of major axis (-222.6187, 300) minor radius 8
  ellipse E193 centre (-204.6187, 268) end of major axis (-222.6187, 268) minor radius 8
  ellipse E194 centre (-204.6187, 236) end of major axis (-222.6187, 236) minor radius 8
  ellipse E195 centre (-204.6187, 204) end of major axis (-222.6187, 204) minor radius 8
  ellipse E196 centre (-204.6187, 172) end of major axis (-222.6187, 172) minor radius 8
  ellipse E197 centre (-204.6187, 140) end of major axis (-222.6187, 140) minor radius 8
  ellipse E198 centre (-204.6187, 428) end of major axis (-222.6187, 428) minor radius 8
  ellipse E199 centre (-204.6187, 396) end of major axis (-222.6187, 396) minor radius 8
  ellipse E200 centre (-204.6187, 364) end of major axis (-222.6187, 364) minor radius 8
  ellipse E201 centre (-204.6187, 332) end of major axis (-222.6187, 332) minor radius 8
  ellipse E202 centre (-204.6187, 300) end of major axis (-222.6187, 300) minor radius 8
  ellipse E203 centre (-204.6187, 268) end of major axis (-222.6187, 268) minor radius 8
  ellipse E204 centre (-204.6187, 236) end of major axis (-222.6187, 236) minor radius 8
  ellipse E205 centre (-204.6187, 204) end of major axis (-222.6187, 204) minor radius 8
  ellipse E206 centre (-204.6187, 172) end of major axis (-222.6187, 172) minor radius 8
  ellipse E207 centre (-204.6187, 460) end of major axis (-222.6187, 460) minor radius 8
  ellipse E208 centre (-204.6187, 428) end of major axis (-222.6187, 428) minor radius 8
  ellipse E209 centre (-204.6187, 396) end of major axis (-222.6187, 396) minor radius 8
  ellipse E210 centre (-204.6187, 364) end of major axis (-222.6187, 364) minor radius 8
  ellipse E211 centre (-204.6187, 332) end of major axis (-222.6187, 332) minor radius 8
  ellipse E212 centre (-204.6187, 300) end of major axis (-222.6187, 300) minor radius 8
  ellipse E213 centre (-204.6187, 268) end of major axis (-222.6187, 268) minor radius 8
  ellipse E214 centre (-204.6187, 236) end of major axis (-222.6187, 236) minor radius 8
  ellipse E215 centre (-204.6187, 204) end of major axis (-222.6187, 204) minor radius 8
  ellipse E216 centre (-204.6187, 492) end of major axis (-222.6187, 492) minor radius 8
  ellipse E217 centre (-204.6187, 460) end of major axis (-222.6187, 460) minor radius 8
  ellipse E218 centre (-204.6187, 428) end of major axis (-222.6187, 428) minor radius 8
  ellipse E219 centre (-204.6187, 396) end of major axis (-222.6187, 396) minor radius 8
  ellipse E220 centre (-204.6187, 364) end of major axis (-222.6187, 364) minor radius 8
  ellipse E221 centre (-204.6187, 332) end of major axis (-222.6187, 332) minor radius 8
  ellipse E222 centre (-204.6187, 300) end of major axis (-222.6187, 300) minor radius 8
  ellipse E223 centre (-204.6187, 268) end of major axis (-222.6187, 268) minor radius 8
  ellipse E224 centre (-204.6187, 236) end of major axis (-222.6187, 236) minor radius 8
  ellipse E225 centre (-204.6187, 524) end of major axis (-222.6187, 524) minor radius 8
  ellipse E226 centre (-204.6187, 492) end of major axis (-222.6187, 492) minor radius 8
  ellipse E227 centre (-204.6187, 460) end of major axis (-222.6187, 460) minor radius 8
  ellipse E228 centre (-204.6187, 428) end of major axis (-222.6187, 428) minor radius 8
  ellipse E229 centre (-204.6187, 396) end of major axis (-222.6187, 396) minor radius 8
  ellipse E230 centre (-204.6187, 364) end of major axis (-222.6187, 364) minor radius 8
  ellipse E231 centre (-204.6187, 332) end of major axis (-222.6187, 332) minor radius 8
  ellipse E232 centre (-204.6187, 300) end of major axis (-222.6187, 300) minor radius 8
  ellipse E233 centre (-204.6187, 268) end of major axis (-222.6187, 268) minor radius 8
  ellipse E234 centre (-204.6187, 556) end of major axis (-222.6187, 556) minor radius 8
  ellipse E235 centre (-204.6187, 524) end of major axis (-222.6187, 524) minor radius 8
  ellipse E236 centre (-204.6187, 492) end of major axis (-222.6187, 492) minor radius 8
  ellipse E237 centre (-204.6187, 460) end of major axis (-222.6187, 460) minor radius 8
  ellipse E238 centre (-204.6187, 428) end of major axis (-222.6187, 428) minor radius 8
  ellipse E239 centre (-204.6187, 396) end of major axis (-222.6187, 396) minor radius 8
  ellipse E240 centre (-204.6187, 364) end of major axis (-222.6187, 364) minor radius 8
  ellipse E241 centre (-204.6187, 332) end of major axis (-222.6187, 332) minor radius 8
  ellipse E242 centre (-204.6187, 300) end of major axis (-222.6187, 300) minor radius 8
  point P0 (385.1344, 600)
  point P1 (33.9946, 292)
  point P2 (33.9946, 308)
  point P3 (33.9946, 260)
  point P4 (33.9946, 276)
  point P5 (33.9946, 228)
  point P6 (33.9946, 244)
  point P7 (33.9946, 196)
  point P8 (33.9946, 212)
  point P9 (33.9946, 164)
  point P10 (33.9946, 180)
  point P11 (33.9946, 132)
  point P12 (33.9946, 148)
  point P13 (33.9946, 100)
  point P14 (33.9946, 116)
  point P15 (33.9946, 68)
  point P16 (33.9946, 84)
  point P17 (33.9946, 36)
  point P18 (33.9946, 52)
  point P19 (33.9946, 324)
  point P20 (33.9946, 340)
  point P21 (33.9946, 292)
  point P22 (33.9946, 308)
  point P23 (33.9946, 260)
  point P24 (33.9946, 276)
  point P25 (33.9946, 228)
  point P26 (33.9946, 244)
  point P27 (33.9946, 196)
  point P28 (33.9946, 212)
  point P29 (33.9946, 164)
  point P30 (33.9946, 180)
  point P31 (33.9946, 132)
  point P32 (33.9946, 148)
  point P33 (33.9946, 100)
  point P34 (33.9946, 116)
  point P35 (33.9946, 68)
  point P36 (33.9946, 84)
  point P37 (33.9946, 356)
  point P38 (33.9946, 372)
  point P39 (33.9946, 324)
  point P40 (33.9946, 340)
  point P41 (33.9946, 292)
  point P42 (33.9946, 308)
  point P43 (33.9946, 260)
  point P44 (33.9946, 276)
  point P45 (33.9946, 228)
  point P46 (33.9946, 244)
  point P47 (33.9946, 196)
  point P48 (33.9946, 212)
  point P49 (33.9946, 164)
  point P50 (33.9946, 180)
  point P51 (33.9946, 132)
  point P52 (33.9946, 148)
  point P53 (33.9946, 100)
  point P54 (33.9946, 116)
  point P55 (33.9946, 388)
  point P56 (33.9946, 404)
  point P57 (33.9946, 356)
  point P58 (33.9946, 372)
  point P59 (33.9946, 324)
  point P60 (33.9946, 340)
  point P61 (33.9946, 292)
  point P62 (33.9946, 308)
  point P63 (33.9946, 260)
  point P64 (33.9946, 276)
  point P65 (33.9946, 228)
  point P66 (33.9946, 244)
  point P67 (33.9946, 196)
  point P68 (33.9946, 212)
  point P69 (33.9946, 164)
  point P70 (33.9946, 180)
  point P71 (33.9946, 132)
  point P72 (33.9946, 148)
  point P73 (33.9946, 420)
  point P74 (33.9946, 436)
  point P75 (33.9946, 388)
  point P76 (33.9946, 404)
  point P77 (33.9946, 356)
  point P78 (33.9946, 372)
  point P79 (33.9946, 324)
  point P80 (33.9946, 340)
  point P81 (33.9946, 292)
  point P82 (33.9946, 308)
  point P83 (33.9946, 260)
  point P84 (33.9946, 276)
  point P85 (33.9946, 228)
  point P86 (33.9946, 244)
  point P87 (33.9946, 196)
  point P88 (33.9946, 212)
  point P89 (33.9946, 164)
  point P90 (33.9946, 180)
  point P91 (33.9946, 452)
  point P92 (33.9946, 468)
  point P93 (33.9946, 420)
  point P94 (33.9946, 436)
  point P95 (33.9946, 388)
  point P96 (33.9946, 404)
  point P97 (33.9946, 356)